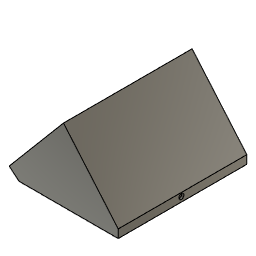
Custom StreamDeck v1 (Autodesk Fusion 360 design; units mm, degrees)
Autodesk Fusion 360 part; units mm, degrees
sketch "Esquisse1" plane through (0, 0, 0) normal (0, 0, 1) x (1, 0, 0)
  line L0 (0.1341, -76.3658) -> (64.4137, -0.1129)
  line L1 (64.4137, -0.1129) -> (129.0708, -76.1647)
  line L2 (129.0708, -76.1647) -> (129.0708, -86.1624)
  line L3 (0.1341, -76.133) -> (11.9451, -86.0425)
  line L4 (129.2084, -85.9931) -> (11.8004, -85.9931)
extrude "Extrusion1" add sketch "Esquisse1" along normal blind 148
move_body "Déplacer1" bodies 1 to x (1, 0, 0) y (0, 0, 1) z (0, -1, 0) at (0, 20.1587, 192.145)
sketch "Esquisse2" plane through (-56.9768, 0, 48.0303) normal (-0.764582, 0, 0.644527) x (0, -1, 0)
  line L0 (-20.1587, 188.3406) -> (-20.1587, 88.7874)
  line L1 (-20.1587, 88.7874) -> (127.8413, 88.7874)
  line L2 (127.8413, 88.7874) -> (127.8413, 188.3406)
  line L3 (127.8413, 188.3406) -> (-20.1587, 188.3406)
  line L4 (-18.8236, 187.8236) -> (126.1751, 187.8236)
  line L5 (126.1751, 187.8236) -> (126.1751, 87.8252)
  line L6 (126.1751, 87.8252) -> (-18.8236, 87.8252)
  line L7 (-18.8236, 87.8252) -> (-18.8236, 187.8236)
  line L8 (-3.8235, 175.0777) -> (11.1766, 175.0777)
  line L9 (11.1766, 175.0777) -> (11.1766, 160.0776)
  line L10 (11.1766, 160.0776) -> (-3.8235, 160.0776)
  line L11 (-3.8235, 160.0776) -> (-3.8235, 175.0777)
  line L12 (21.1779, 175.0777) -> (36.178, 175.0777)
  line L13 (36.178, 175.0777) -> (36.178, 160.0776)
  line L14 (36.178, 160.0776) -> (21.1779, 160.0776)
  line L15 (21.1779, 160.0776) -> (21.1779, 175.0777)
  line L16 (46.1757, 175.0777) -> (61.1758, 175.0777)
  line L17 (61.1758, 175.0777) -> (61.1758, 160.0776)
  line L18 (61.1758, 160.0776) -> (46.1757, 160.0776)
  line L19 (46.1757, 160.0776) -> (46.1757, 175.0777)
  line L20 (71.1771, 175.0777) -> (86.1772, 175.0777)
  line L21 (86.1772, 175.0777) -> (86.1772, 160.0776)
  line L22 (86.1772, 160.0776) -> (71.1771, 160.0776)
  line L23 (71.1771, 160.0776) -> (71.1771, 175.0777)
  line L24 (96.1749, 175.0777) -> (111.175, 175.0777)
  line L25 (111.175, 175.0777) -> (111.175, 160.0776)
  line L26 (111.175, 160.0776) -> (96.1749, 160.0776)
  line L27 (96.1749, 160.0776) -> (96.1749, 175.0777)
  line L28 (-3.8235, 155.1387) -> (11.1766, 155.1387)
  line L29 (11.1766, 155.1387) -> (11.1766, 140.1386)
  line L30 (11.1766, 140.1386) -> (-3.8235, 140.1386)
  line L31 (-3.8235, 140.1386) -> (-3.8235, 155.1387)
  line L32 (21.1779, 155.1387) -> (36.178, 155.1387)
  line L33 (36.178, 155.1387) -> (36.178, 140.1386)
  line L34 (36.178, 140.1386) -> (21.1779, 140.1386)
  line L35 (21.1779, 140.1386) -> (21.1779, 155.1387)
  line L36 (46.1757, 155.1387) -> (61.1758, 155.1387)
  line L37 (61.1758, 155.1387) -> (61.1758, 140.1386)
  line L38 (61.1758, 140.1386) -> (46.1757, 140.1386)
  line L39 (46.1757, 140.1386) -> (46.1757, 155.1387)
  line L40 (71.1771, 155.1387) -> (86.1772, 155.1387)
  line L41 (86.1772, 155.1387) -> (86.1772, 140.1386)
  line L42 (86.1772, 140.1386) -> (71.1771, 140.1386)
  line L43 (71.1771, 140.1386) -> (71.1771, 155.1387)
  line L44 (96.1749, 155.1387) -> (111.175, 155.1387)
  line L45 (111.175, 155.1387) -> (111.175, 140.1386)
  line L46 (111.175, 140.1386) -> (96.1749, 140.1386)
  line L47 (96.1749, 140.1386) -> (96.1749, 155.1387)
  line L48 (-3.8235, 135.1997) -> (11.1766, 135.1997)
  line L49 (11.1766, 135.1997) -> (11.1766, 120.1996)
  line L50 (11.1766, 120.1996) -> (-3.8235, 120.1996)
  line L51 (-3.8235, 120.1996) -> (-3.8235, 135.1997)
  line L52 (21.1779, 135.1997) -> (36.178, 135.1997)
  line L53 (36.178, 135.1997) -> (36.178, 120.1996)
  line L54 (36.178, 120.1996) -> (21.1779, 120.1996)
  line L55 (21.1779, 120.1996) -> (21.1779, 135.1997)
  line L56 (46.1757, 135.1997) -> (61.1758, 135.1997)
  line L57 (61.1758, 135.1997) -> (61.1758, 120.1996)
  line L58 (61.1758, 120.1996) -> (46.1757, 120.1996)
  line L59 (46.1757, 120.1996) -> (46.1757, 135.1997)
  line L60 (71.1771, 135.1997) -> (86.1772, 135.1997)
  line L61 (86.1772, 135.1997) -> (86.1772, 120.1996)
  line L62 (86.1772, 120.1996) -> (71.1771, 120.1996)
  line L63 (71.1771, 120.1996) -> (71.1771, 135.1997)
  line L64 (96.1749, 135.1997) -> (111.175, 135.1997)
  line L65 (111.175, 135.1997) -> (111.175, 120.1996)
  line L66 (111.175, 120.1996) -> (96.1749, 120.1996)
  line L67 (96.1749, 120.1996) -> (96.1749, 135.1997)
  line L68 (-3.8235, 115.2643) -> (11.1766, 115.2643)
  line L69 (11.1766, 115.2643) -> (11.1766, 100.2642)
  line L70 (11.1766, 100.2642) -> (-3.8235, 100.2642)
  line L71 (-3.8235, 100.2642) -> (-3.8235, 115.2643)
  line L72 (21.1779, 115.2643) -> (36.178, 115.2643)
  line L73 (36.178, 115.2643) -> (36.178, 100.2642)
  line L74 (36.178, 100.2642) -> (21.1779, 100.2642)
  line L75 (21.1779, 100.2642) -> (21.1779, 115.2643)
  line L76 (46.1757, 115.2643) -> (61.1758, 115.2643)
  line L77 (61.1758, 115.2643) -> (61.1758, 100.2642)
  line L78 (61.1758, 100.2642) -> (46.1757, 100.2642)
  line L79 (46.1757, 100.2642) -> (46.1757, 115.2643)
  line L80 (71.1771, 115.2643) -> (86.1772, 115.2643)
  line L81 (86.1772, 115.2643) -> (86.1772, 100.2642)
  line L82 (86.1772, 100.2642) -> (71.1771, 100.2642)
  line L83 (71.1771, 100.2642) -> (71.1771, 115.2643)
  line L84 (96.1749, 115.2643) -> (111.175, 115.2643)
  line L85 (111.175, 115.2643) -> (111.175, 100.2642)
  line L86 (111.175, 100.2642) -> (96.1749, 100.2642)
  line L87 (96.1749, 100.2642) -> (96.1749, 115.2643)
shell "Coque1" thickness 2.5 removed faces 1 at (68.4569, -127.8413, 138.0547)
extrude "Extrusion2" cut sketch "Esquisse2" against normal blind 10 contours L8 L9 L10 L11 | L12 L13 L14 L15 | L16 L17 L18 L19 | L20 L21 L22 L23 | L24 L25 L26 L27 | L28 L29 L30 L31 | L32 L33 L34 L35 | L36 L37 L38 L39 | L40 L41 L42 L43 | L44 L45 L46 L47 | L48 L49 L50 L51 | L52 L53 L54 L55 | L56 L57 L58 L59 | L60 L61 L62 L63 | L64 L65 L66 L67 | L68 L69 L70 L71 | L72 L73 L74 L75 | L76 L77 L78 L79 | L80 L81 L82 L83 | L84 L85 L86 L87
hole "Perçage1" at (126.5708, -55.0913, 111.8565) direction (1, 0, 0) diameter 6 depth 60 tip angle 118
sketch "Esquisse3" plane through (0, -127.8413, 0) normal (0, -1, 0) x (1, 0, 0)
  line L0 (3.7755, 116.2201) -> (64.4218, 188.1629)
  line L1 (64.4218, 188.1629) -> (126.5708, 115.0612)
  line L2 (126.5708, 115.0612) -> (126.5708, 108.6519)
  line L3 (126.5708, 108.6519) -> (12.796, 108.6519)
  line L4 (12.796, 108.6519) -> (3.7755, 116.2201)
  line L5 (0.249, 115.9156) -> (11.8862, 106.1519)
  line L6 (11.8862, 106.1519) -> (129.0708, 106.1519)
  line L7 (129.0708, 106.1519) -> (129.0708, 115.9803)
  line L8 (129.0708, 115.9803) -> (64.4137, 192.0321)
  line L9 (64.4137, 192.0321) -> (0.249, 115.9156)
  line L10 (64.4137, 192.0321) -> (0.249, 115.9156)
  line L11 (11.8862, 106.1519) -> (129.0708, 106.1519)
  line L12 (129.0708, 115.9803) -> (64.4137, 192.0321)
  constraint coincident L8.end L9.start
  constraint coincident L5.start L9.end
  constraint coincident L5.end L6.start
  constraint coincident L6.end L7.start
  constraint coincident L7.end L8.start
extrude "Extrusion3" add sketch "Esquisse3" along normal blind 2 contours L0 L1 L2 L3 L4 | L5 L6 L7 L8 L9 L10 L11 L12
move_face "DécalerLesFaces1" offset 2 1 faces at (68.4569, 20.1587, 138.0547)
